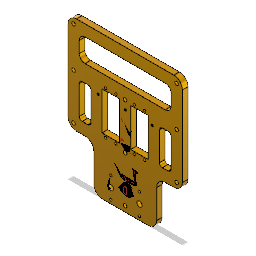
grt_lower_torso_20190218 (Autodesk Fusion 360 design; units mm, degrees)
Autodesk Fusion 360 part; units mm, degrees
sketch "Skizze1" plane through (0, 0, 0) normal (0, 0, 1) x (1, 0, 0)
  circle A0 centre (-25, -56.5195) radius 2.05
  circle A1 centre (-25, -93.5195) radius 2.05
  circle A2 centre (-25, -75.0195) radius 4.5
  circle A3 centre (25, -93.5195) radius 2.05
  circle A4 centre (25, -56.5195) radius 2.05
  circle A5 centre (25, -75.0195) radius 4.5
  line L0 (40, -100.0195) -> (-40, -100.0195)
  line L1 (-55, -85.0195) -> (-55, -35.0195)
  line L2 (-70, -20.0195) -> (-85, -20.0195)
  line L3 (-100, -5.0195) -> (-100, 134.9805)
  line L4 (-85, 149.9805) -> (85, 149.9805)
  line L5 (100, 134.9805) -> (100, -5.0195)
  line L6 (85, -20.0195) -> (70, -20.0195)
  line L7 (55, -35.0195) -> (55, -85.0195)
  line L8 (70, 129.9805) -> (-70, 129.9805)
  line L9 (-80, 119.9805) -> (-80, 99.9805)
  line L10 (-70, 89.9805) -> (70, 89.9805)
  line L11 (80, 99.9805) -> (80, 119.9805)
  line L12 (9.75, -0.0695) -> (40.25, -0.0695)
  line L13 (40.25, 66.4305) -> (9.75, 66.4305)
  circle A6 centre (34, 70.6805) radius 2.05
  circle A7 centre (34, -4.3195) radius 2.05
  line L14 (40.25, -0.0695) -> (40.25, 66.4305)
  circle A8 centre (16, -4.3195) radius 2.05
  line L15 (9.75, 66.4305) -> (9.75, -0.0695)
  circle A9 centre (16, 70.6805) radius 2.05
  line L16 (-40.25, -0.0695) -> (-9.75, -0.0695)
  line L17 (-9.75, 66.4305) -> (-40.25, 66.4305)
  circle A10 centre (-16, 70.6805) radius 2.05
  circle A11 centre (-16, -4.3195) radius 2.05
  line L18 (-9.75, -0.0695) -> (-9.75, 66.4305)
  circle A12 centre (-34, -4.3195) radius 2.05
  line L19 (-40.25, 66.4305) -> (-40.25, -0.0695)
  circle A13 centre (-34, 70.6805) radius 2.05
  arc A14 (100, 134.9805) -> (85, 149.9805) centre (85, 134.9805) ccw
  arc A15 (-85, 149.9805) -> (-100, 134.9805) centre (-85, 134.9805) ccw
  arc A16 (-100, -5.0195) -> (-85, -20.0195) centre (-85, -5.0195) ccw
  arc A17 (85, -20.0195) -> (100, -5.0195) centre (85, -5.0195) ccw
  arc A18 (40, -100.0195) -> (55, -85.0195) centre (40, -85.0195) ccw
  arc A19 (-55, -85.0195) -> (-40, -100.0195) centre (-40, -85.0195) ccw
  arc A20 (-55, -35.0195) -> (-70, -20.0195) centre (-70, -35.0195) ccw
  arc A21 (70, -20.0195) -> (55, -35.0195) centre (70, -35.0195) ccw
  line L20 (-75, 59.9805) -> (-65, 59.9805)
  line L21 (-60, 54.9805) -> (-60, 4.9805)
  line L22 (-65, -0.0195) -> (-75, -0.0195)
  line L23 (-80, 4.9805) -> (-80, 54.9805)
  arc A22 (-80, 99.9805) -> (-70, 89.9805) centre (-70, 99.9805) ccw
  arc A23 (-70, 129.9805) -> (-80, 119.9805) centre (-70, 119.9805) ccw
  arc A24 (70, 89.9805) -> (80, 99.9805) centre (70, 99.9805) ccw
  arc A25 (80, 119.9805) -> (70, 129.9805) centre (70, 119.9805) ccw
  arc A26 (-60, 54.9805) -> (-65, 59.9805) centre (-65, 54.9805) ccw
  arc A27 (-75, 59.9805) -> (-80, 54.9805) centre (-75, 54.9805) ccw
  arc A28 (-80, 4.9805) -> (-75, -0.0195) centre (-75, 4.9805) ccw
  arc A29 (-65, -0.0195) -> (-60, 4.9805) centre (-65, 4.9805) ccw
  line L24 (75, 59.9805) -> (65, 59.9805)
  line L25 (60, 54.9805) -> (60, 4.9805)
  line L26 (65, -0.0195) -> (75, -0.0195)
  line L27 (80, 4.9805) -> (80, 54.9805)
  arc A30 (80, 54.9805) -> (75, 59.9805) centre (75, 54.9805) ccw
  arc A31 (65, 59.9805) -> (60, 54.9805) centre (65, 54.9805) ccw
  arc A32 (60, 4.9805) -> (65, -0.0195) centre (65, 4.9805) ccw
  arc A33 (75, -0.0195) -> (80, 4.9805) centre (75, 4.9805) ccw
  circle A34 centre (90, 69.9805) radius 3.05
  circle A35 centre (-90, 69.9805) radius 3.05
  circle A36 centre (90, 139.9805) radius 3.05
  circle A37 centre (-90, 139.9805) radius 3.05
  circle A38 centre (90, -10) radius 3.05
  circle A39 centre (-90, -10) radius 3.05
  circle A40 centre (0, 69.9805) radius 3.05
  circle A41 centre (0, -90.0195) radius 3.05
  circle A42 centre (0, -10) radius 3.05
  dimension "d5" = 9
  dimension "d6" = 4.1
  dimension "d7" = 18.5
  dimension "d8" = 4.1
  dimension "d9" = 18.5
  dimension "d10" = 9
  dimension "d11" = 4.1
  dimension "d12" = 18.5
  dimension "d13" = 4.1
  dimension "d14" = 18.5
  dimension "d15" = 25
  dimension "d16" = 200
  dimension "d18" = 25
  dimension "d47" = 25
  dimension "d68" = 15.25
  dimension "d69" = 15.25
  dimension "d70" = 33.25
  dimension "d71" = 33.25
  dimension "d72" = 4.1
  dimension "d73" = 18
  dimension "d74" = 75
  dimension "d78" = 15.25
  dimension "d79" = 15.25
  dimension "d80" = 15.25
  dimension "d81" = 33.25
  dimension "d82" = 33.25
  dimension "d83" = 4.1
  dimension "d84" = 18
  dimension "d85" = 75
  dimension "d89" = 15.25
  dimension "d90" = 9
  dimension "d91" = 37.5
  dimension "d94" = 25
  dimension "d95" = 25
  dimension "d98" = 37.5
  dimension "d99" = 9
  dimension "d100" = 15
  dimension "d101" = 15
  dimension "d104" = 20
  dimension "d105" = 20
  dimension "d106" = 20
  dimension "d107" = 40
  dimension "d108" = 10
  dimension "d109" = 5
  dimension "d110" = 5
  dimension "d113" = 55
  dimension "d114" = 55
  dimension "d115" = 250
  dimension "d116" = 170
  dimension "d117" = 20
  dimension "d118" = 20
  dimension "d120" = 20
  dimension "d121" = 60
  dimension "d122" = 170
  dimension "d123" = 20
  dimension "d124" = 20
  dimension "d125" = 60
  dimension "d126" = 20
  dimension "d127" = 6.1
  dimension "d128" = 10
  dimension "d129" = 10
  dimension "d130" = 10
  dimension "d131" = 10
  dimension "d132" = 10
  dimension "d133" = 10
  dimension "d134" = 10
  dimension "d135" = 10
  dimension "d136" = 10
  dimension "d137" = 10
  dimension "d139" = 100
  dimension "d194" = 18.2
  dimension "d195" = 18.2
  dimension "d197" = 90
  dimension "d198" = 90
  measures "d5" diameter of A2
  measures "d6" diameter of A1
  measures "d8" diameter of A0
  measures "d10" diameter of A5
  measures "d11" diameter of A4
  measures "d13" diameter of A3
  measures "d68" distance of origin L14
  measures "d69" distance of origin L15
  measures "d70" distance of origin L13
  measures "d71" distance of origin L12
  measures "d72" diameter of A6
  measures "d73" distance of origin
  measures "d74" distance of origin
  measures "d78" distance of L14
  measures "d79" distance of origin L18
  measures "d80" distance of origin L19
  measures "d81" distance of origin L17
  measures "d82" distance of origin L16
  measures "d83" diameter of A10
  measures "d84" distance of origin
  measures "d89" distance of L18
  measures "d98" distance of origin
  measures "d99" distance of origin
  measures "d100" radius of A14
  measures "d101" radius of A15
  measures "d104" distance of L4 L8
  measures "d105" distance of L3 L9
  measures "d106" distance of L5 L11
  measures "d107" distance of L8 L10
  measures "d108" radius of A22
  measures "d109" radius of A26
  measures "d110" radius of A30
  measures "d115" distance of L0 L4
  measures "d116" distance of L2 L4
  measures "d117" distance of L2 L22
  measures "d118" distance of L3 L23
  measures "d120" distance of L21 L23
  measures "d121" distance of L20 L22
  measures "d122" distance of L4 L6
  measures "d123" distance of L5 L27
  measures "d124" distance of L25 L27
  measures "d125" distance of L24 L26
  measures "d126" distance of L6 L26
  measures "d127" diameter of A34
  measures "d128" distance of L5 origin
  measures "d130" distance of L3 origin
  measures "d132" distance of L5 origin
  measures "d134" distance of L3 origin
  measures "d137" distance of origin
  measures "d139" distance of L3 origin
  measures "d194" distance of origin
  measures "d195" distance of origin
  measures "d197" distance of origin
  measures "d198" distance of origin
extrude "Extrusion3" add sketch "Skizze1" along normal blind 10
sketch "Skizze2" plane through (0, 0, 10) normal (0, 0, 1) x (1, 0, 0)
  circle A0 centre (-90, 69.9805) radius 3.05
  circle A1 centre (0, -90.0195) radius 3.05
  circle A2 centre (0, -10) radius 3.05
  circle A3 centre (0, 69.9805) radius 3.05
  circle A4 centre (-90, -10) radius 3.05
  circle A5 centre (90, -10) radius 3.05
  circle A6 centre (-90, 139.9805) radius 3.05
  circle A7 centre (90, 139.9805) radius 3.05
  circle A8 centre (-25, -93.5195) radius 2.05
  circle A9 centre (-25, -75.0195) radius 4.5
  circle A10 centre (25, -93.5195) radius 2.05
  circle A11 centre (16, 70.6805) radius 2.05
  circle A12 centre (-16, 70.6805) radius 2.05
  arc A13 (75, -0.0195) -> (80, 4.9805) centre (75, 4.9805) ccw
  line L0 (75, -0.0195) -> (65, -0.0195)
  arc A14 (60, 4.9805) -> (65, -0.0195) centre (65, 4.9805) ccw
  line L1 (60, 4.9805) -> (60, 54.9805)
  arc A15 (65, 59.9805) -> (60, 54.9805) centre (65, 54.9805) ccw
  line L2 (65, 59.9805) -> (75, 59.9805)
  arc A16 (80, 54.9805) -> (75, 59.9805) centre (75, 54.9805) ccw
  line L3 (80, 54.9805) -> (80, 4.9805)
  circle A17 centre (-16, -4.3195) radius 2.05
  circle A18 centre (90, 69.9805) radius 3.05
  circle A19 centre (-25, -56.5195) radius 2.05
  circle A20 centre (-34, 70.6805) radius 2.05
  line L4 (-40.25, -0.0695) -> (-40.25, 66.4305)
  line L5 (-40.25, 66.4305) -> (-9.75, 66.4305)
  line L6 (-9.75, 66.4305) -> (-9.75, -0.0695)
  line L7 (-9.75, -0.0695) -> (-40.25, -0.0695)
  circle A21 centre (-34, -4.3195) radius 2.05
  arc A22 (-80, 4.9805) -> (-75, -0.0195) centre (-75, 4.9805) ccw
  line L8 (-80, 4.9805) -> (-80, 54.9805)
  arc A23 (-75, 59.9805) -> (-80, 54.9805) centre (-75, 54.9805) ccw
  line L9 (-75, 59.9805) -> (-65, 59.9805)
  arc A24 (-60, 54.9805) -> (-65, 59.9805) centre (-65, 54.9805) ccw
  line L10 (-60, 54.9805) -> (-60, 4.9805)
  arc A25 (-65, -0.0195) -> (-60, 4.9805) centre (-65, 4.9805) ccw
  line L11 (-65, -0.0195) -> (-75, -0.0195)
  arc A26 (80, 119.9805) -> (70, 129.9805) centre (70, 119.9805) ccw
  line L12 (80, 119.9805) -> (80, 99.9805)
  arc A27 (70, 89.9805) -> (80, 99.9805) centre (70, 99.9805) ccw
  line L13 (70, 89.9805) -> (-70, 89.9805)
  arc A28 (-80, 99.9805) -> (-70, 89.9805) centre (-70, 99.9805) ccw
  line L14 (-80, 99.9805) -> (-80, 119.9805)
  arc A29 (-70, 129.9805) -> (-80, 119.9805) centre (-70, 119.9805) ccw
  line L15 (-70, 129.9805) -> (70, 129.9805)
  circle A30 centre (34, 70.6805) radius 2.05
  circle A31 centre (25, -56.5195) radius 2.05
  circle A32 centre (16, -4.3195) radius 2.05
  circle A33 centre (25, -75.0195) radius 4.5
  circle A34 centre (34, -4.3195) radius 2.05
  line L16 (9.75, -0.0695) -> (9.75, 66.4305)
  line L17 (9.75, 66.4305) -> (40.25, 66.4305)
  line L18 (40.25, 66.4305) -> (40.25, -0.0695)
  line L19 (40.25, -0.0695) -> (9.75, -0.0695)
  arc A35 (85, -20.0195) -> (100, -5.0195) centre (85, -5.0195) ccw
  line L20 (100, -5.0195) -> (100, 134.9805)
  arc A36 (100, 134.9805) -> (85, 149.9805) centre (85, 134.9805) ccw
  line L21 (85, 149.9805) -> (-85, 149.9805)
  arc A37 (-85, 149.9805) -> (-100, 134.9805) centre (-85, 134.9805) ccw
  line L22 (-100, 134.9805) -> (-100, -5.0195)
  arc A38 (-100, -5.0195) -> (-85, -20.0195) centre (-85, -5.0195) ccw
  line L23 (-85, -20.0195) -> (-70, -20.0195)
  arc A39 (-55, -35.0195) -> (-70, -20.0195) centre (-70, -35.0195) ccw
  line L24 (-55, -35.0195) -> (-55, -85.0195)
  arc A40 (-55, -85.0195) -> (-40, -100.0195) centre (-40, -85.0195) ccw
  line L25 (-40, -100.0195) -> (40, -100.0195)
  arc A41 (40, -100.0195) -> (55, -85.0195) centre (40, -85.0195) ccw
  line L26 (55, -85.0195) -> (55, -35.0195)
  arc A42 (70, -20.0195) -> (55, -35.0195) centre (70, -35.0195) ccw
  line L27 (70, -20.0195) -> (85, -20.0195)
  line L28 (85, -20.0195) -> (70, -20.0195)
  line L29 (100, 134.9805) -> (100, -5.0195)
  line L30 (-70, -20.0195) -> (-85, -20.0195)
  line L31 (-100, -5.0195) -> (-100, 134.9805)
  line L32 (60, 54.9805) -> (60, 4.9805)
  line L33 (-60, 54.9805) -> (-60, 4.9805)
  line L34 (-48.25, 56.4305) -> (-46.25, 56.4305)
  line L35 (-45.75, 55.9305) -> (-45.75, 53.9305)
  line L36 (-46.25, 53.4305) -> (-48.25, 53.4305)
  line L37 (-48.75, 53.9305) -> (-48.75, 55.9305)
  arc A43 (-48.25, 56.4305) -> (-48.75, 55.9305) centre (-48.25, 55.9305) ccw
  arc A44 (-45.75, 55.9305) -> (-46.25, 56.4305) centre (-46.25, 55.9305) ccw
  arc A45 (-46.25, 53.4305) -> (-45.75, 53.9305) centre (-46.25, 53.9305) ccw
  arc A46 (-48.75, 53.9305) -> (-48.25, 53.4305) centre (-48.25, 53.9305) ccw
  line L38 (-40.25, 66.4305) -> (-40.25, -0.0695)
  line L39 (-9.75, 66.4305) -> (-40.25, 66.4305)
  line L40 (48.75, 55.9305) -> (48.75, 53.9305)
  arc A47 (46.25, 56.4305) -> (45.75, 55.9305) centre (46.25, 55.9305) ccw
  arc A48 (48.25, 53.4305) -> (48.75, 53.9305) centre (48.25, 53.9305) ccw
  arc A49 (45.75, 53.9305) -> (46.25, 53.4305) centre (46.25, 53.9305) ccw
  line L41 (48.25, 53.4305) -> (46.25, 53.4305)
  line L42 (46.25, 56.4305) -> (48.25, 56.4305)
  line L43 (45.75, 53.9305) -> (45.75, 55.9305)
  arc A50 (48.75, 55.9305) -> (48.25, 56.4305) centre (48.25, 55.9305) ccw
  line L44 (40.25, -0.0695) -> (40.25, 66.4305)
  line L45 (40.25, 66.4305) -> (9.75, 66.4305)
  line L46 (1.75, 55.9305) -> (1.75, 53.9305)
  arc A51 (-0.75, 56.4305) -> (-1.25, 55.9305) centre (-0.75, 55.9305) ccw
  arc A52 (1.25, 53.4305) -> (1.75, 53.9305) centre (1.25, 53.9305) ccw
  arc A53 (-1.25, 53.9305) -> (-0.75, 53.4305) centre (-0.75, 53.9305) ccw
  line L47 (1.25, 53.4305) -> (-0.75, 53.4305)
  line L48 (-0.75, 56.4305) -> (1.25, 56.4305)
  line L49 (-1.25, 53.9305) -> (-1.25, 55.9305)
  arc A54 (1.75, 55.9305) -> (1.25, 56.4305) centre (1.25, 55.9305) ccw
  line L50 (9.75, 66.4305) -> (9.75, -0.0695)
  point P0 (-20, 0)
  point P1 (-20, 0)
  dimension "d177" = 3
  dimension "d178" = 3
  dimension "d179" = 0.5
  dimension "d180" = 5.5
  dimension "d181" = 10
  dimension "d182" = 3
  dimension "d183" = 3
  dimension "d184" = 0.5
  dimension "d185" = 5.5
  dimension "d186" = 10
  dimension "d187" = 3
  dimension "d188" = 3
  dimension "d189" = 0.5
  dimension "d190" = 8
  dimension "d191" = 10
  measures "d179" radius of A43
  measures "d180" distance of L35 L38
  measures "d181" distance of L34 L39
  measures "d184" radius of A47
  measures "d185" distance of L43 L44
  measures "d186" distance of L42 L45
  measures "d187" distance of P1
  measures "d189" radius of A51
  measures "d190" distance of L46 L50
  measures "d191" distance of L45 L48
extrude "Extrusion5" cut sketch "Skizze2" against normal blind 10 contours L34 L35 L36 L37 A43 A44 A45 A46 | L40 A47 A48 A49 L41 L42 L43 A50 | L46 A51 A52 A53 L47 L48 L49 A54
equation "d68 = 15 mm + tolerance"
equation "d69 = 15 mm + tolerance"
equation "d70 = 33 mm + tolerance"
equation "d71 = 33 mm + tolerance"
equation "d78 = 15 mm + tolerance"
equation "d79 = 15 mm + tolerance"
equation "d80 = 15 mm + tolerance"
equation "d81 = 33 mm + tolerance"
equation "d82 = 33 mm + tolerance"
equation "d89 = 15 mm + tolerance"
equation "tolerance = 0.25 mm"
named bodies: "Body2"
